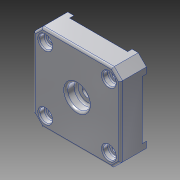
# Autodesk Inventor part: Nema 17 Base
Saved by Autodesk Inventor 2016 (Build 200138000, 138)
## iProperties
Created: 2015-09-21
Part Number: Nema 17 Base
Material: Aluminum 6061
Document SubType Name: Modeling
Designer: Dr Kreigar
Density: 2.7 g/cm^3
Appearance: Aluminum - Flat
Author: Dr Kreigar
Autodesk Inventor part; units mm, degrees
ref_plane "YZ Plane" through (0, 0, 0) normal (1, 0, 0) x (0, 1, 0)
ref_plane "XZ Plane" through (0, 0, 0) normal (0, 1, 0) x (-1, 0, 0)
ref_plane "XY Plane" through (0, 0, 0) normal (0, 0, 1) x (1, 0, 0)
sketch "Sketch1" plane through (0, 0, 0) normal (0, 1, 0) x (-1, 0, 0)
  line L0 (0, 0) -> (-42.3, 0)
  line L1 (-42.3, 0) -> (-42.3, -42.3)
  line L2 (-42.3, -42.3) -> (0, -42.3)
  line L3 (0, -42.3) -> (0, 0)
  dimension "d0" = 42.3
  dimension "d1" = 42.3
  constraints: 8 end point, 2 parallel, 1 horizontal, 1 perpendicular
  measures "d0" distance of L2.end L1.end
  measures "d1" distance of L1.end L0.end
extrude "Extrusion1" add sketch "Sketch1" along normal blind 10.5
sketch "Sketch2" plane through (0, 10.5, 0) normal (0, 1, 0) x (1, 0, 0)
  line L0 (4.0001, 0) -> (0, 4.0001)
  line L1 (0, 42.3) -> (0, 0) construction
  line L2 (0, 0) -> (42.3, 0) construction
  line L3 (42.3, 42.3) -> (0, 42.3) construction
  line L4 (21.15, 42.3) -> (21.15, 0) construction
  line L5 (0, 21.15) -> (42.3, 21.15) construction
  line L6 (42.3, 0) -> (42.3, 42.3) construction
  line L7 (38.2999, 0) -> (42.3, 4.0001)
  line L8 (4.0001, 42.3) -> (0, 38.2999)
  line L9 (38.2999, 42.3) -> (42.3, 38.2999)
  line L10 (0, 4.0001) -> (0, 0)
  line L11 (4.0001, 0) -> (0, 0)
  line L12 (42.3, 4.0001) -> (42.3, 0)
  line L13 (38.2999, 0) -> (42.3, 0)
  line L14 (0, 38.2999) -> (0, 42.3)
  line L15 (4.0001, 42.3) -> (0, 42.3)
  line L16 (42.3, 38.2999) -> (42.3, 42.3)
  line L17 (38.2999, 42.3) -> (42.3, 42.3)
  dimension "d4" = 5.657
  dimension "d5" = 135
  constraints: 28 end point, 6 symmetric about line, 4 midpoint, 2 collinear, 1 point on line
  measures "d4" distance of L0.start L0.end
  measures "d5" angle of L2 L0
extrude "Extrusion2" cut sketch "Sketch2" against normal through all
sketch "Sketch3" plane through (0, 10.5, 0) normal (0, 1, 0) x (1, 0, 0)
  line L0 (0, 38.2999) -> (0, 4.0001) construction
  line L1 (0, 6.9997) -> (6.9997, 0)
  line L2 (4.0001, 0) -> (38.2999, 0) construction
  line L3 (0, 4.0001) -> (4.0001, 0) construction
  line L4 (38.2999, 42.3) -> (4.0001, 42.3) construction
  line L5 (21.15, 42.3) -> (21.15, 0) construction
  line L6 (0, 21.15) -> (42.3, 21.15) construction
  line L7 (42.3, 4.0001) -> (42.3, 38.2999) construction
  line L8 (42.3, 6.9997) -> (35.3003, 0)
  line L9 (0, 35.3003) -> (6.9997, 42.3)
  line L10 (42.3, 35.3003) -> (35.3003, 42.3)
  line L11 (4.0001, 42.3) -> (0, 38.2999) construction
  line L12 (42.3, 38.2999) -> (38.2999, 42.3) construction
  line L13 (38.2999, 0) -> (42.3, 4.0001) construction
  line L14 (0, 35.3003) -> (0, 38.2999)
  line L15 (4.0001, 42.3) -> (6.9997, 42.3)
  line L16 (0, 38.2999) -> (4.0001, 42.3)
  line L17 (38.2999, 42.3) -> (42.3, 38.2999) construction
  line L18 (42.3, 35.3003) -> (42.3, 38.2999)
  line L19 (38.2999, 42.3) -> (35.3003, 42.3)
  line L20 (42.3, 38.2999) -> (38.2999, 42.3)
  line L21 (4.0001, 0) -> (0, 4.0001) construction
  line L22 (42.3, 4.0001) -> (38.2999, 0) construction
  line L23 (0, 6.9997) -> (0, 4.0001)
  line L24 (4.0001, 0) -> (6.9997, 0)
  line L25 (0, 4.0001) -> (4.0001, 0)
  line L26 (42.3, 6.9997) -> (42.3, 4.0001)
  line L27 (38.2999, 0) -> (42.3, 4.0001) construction
  line L28 (42.3, 4.0001) -> (38.2999, 0)
  line L29 (38.2999, 0) -> (35.3003, 0)
  point P0 (0, 0)
  dimension "d8" = 2.121
  constraints: 44 end point, 6 symmetric about line, 4 midpoint, 2 point on line, 1 parallel, 1 perpendicular
  measures "d8" distance between parallel lines of L1 L3
extrude "Extrusion3" add sketch "Sketch3" along normal blind 2.121
hole "Hole1" at (21.15, 10.5, -21.15) direction (0, -1, 0) diameter 5 end through all
hole "Hole2" at (5.65, 10.5, -36.65) direction (0, -1, 0) diameter 3 end through all
pattern_linear "Rectangular Pattern1" count 2 spacing 31 along (1, 0, 0) count 2 spacing 31 along (0, 0, 1) of "Hole2"
hole "Hole3" at (21.15, 0, -21.15) direction (0, 1, 0) diameter 11 depth 5
hole "Hole4" at (36.65, 0, -36.65) direction (0, 1, 0) diameter 6.2 depth 3
pattern_linear "Rectangular Pattern2" count 2 spacing 31 along (-1, 0, 0) count 2 spacing 31 along (0, 0, 1) of "Hole4"
fillet "Fillet1" radius 1 8 edges at (40.2999, 0, -2.0001) (21.15, 0, 0) (2.0001, 0, -2.0001) (0, 0, -21.15) (2.0001, 0, -40.2999) (21.15, 0, -42.3) (40.2999, 0, -40.2999) (42.3, 0, -21.15)
fillet "Fillet2" radius 0.5 8 edges at (36.65, 0, -2.55) (36.65, 3, -2.55) (36.65, 0, -33.55) (36.65, 3, -33.55) (5.65, 0, -33.55) (5.65, 3, -33.55) (5.65, 0, -2.55) (5.65, 3, -2.55)
fillet "Fillet3" radius 1 2 edges at (21.15, 0, -15.65) (21.15, 5, -15.65)
body "Solid1"
